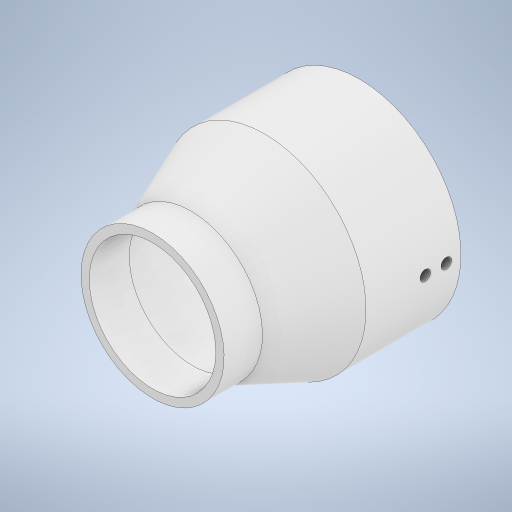
# Autodesk Inventor part: 2in to 4in Reducer
Saved by Autodesk Inventor 2023 (Build 270158030, 158C)
## iProperties
Created: 2022-10-01
Part Number: 2in to 4in Reducer
Material: PVC-Piping
Document SubType Name: Modeling
Designer: cjj5381
Density: 1.4 g/cm^3
Appearance: Smooth - White
Author: cjj5381
Autodesk Inventor part; units mm, degrees
ref_plane "YZ Plane" through (0, 0, 0) normal (1, 0, 0) x (0, 1, 0)
ref_plane "XZ Plane" through (0, 0, 0) normal (0, 1, 0) x (-1, 0, 0)
ref_plane "XY Plane" through (0, 0, 0) normal (0, 0, 1) x (1, 0, 0)
sketch "Sketch1" plane through (0, 0, 0) normal (1, 0, 0) x (0, 1, 0)
  line L0 (30.1625, 50.8) -> (30.1625, 31.75)
  line L1 (30.1625, 31.75) -> (44.45, -3.302)
  line L2 (44.45, -3.302) -> (44.45, -47.752)
  line L3 (0, 0) -> (0, 58.5884)
  line L4 (34.0741, 50.8) -> (34.0741, 32.5166)
  line L5 (34.0741, 32.5166) -> (48.3616, -2.5354)
  line L6 (48.3616, -2.5354) -> (48.3616, -47.752)
  line L7 (34.0741, 50.8) -> (30.1625, 50.8)
  line L8 (48.3616, -47.752) -> (44.45, -47.752)
  line L9 (0, 0) -> (18.7543, 0) construction
  dimension "d0" = 60.325
  dimension "d1" = 88.9
  dimension "d2" = 19.05
  dimension "d3" = 44.45
  dimension "d4" = 3.9116
  dimension "d5" = 98.552
  dimension "d6" = 50.8
  constraints: 20 end point, 3 parallel, 2 horizontal, 2 vertical, 2 other
  measures "d0" diameter of L0 L3
  measures "d1" diameter of L2 L3
  measures "d2" distance of L0.start L0.end
  measures "d3" distance of L1.end L2.end
  measures "d4" distance between parallel lines of L0 L4
  measures "d5" vertical distance of L2.end L0.start
  measures "d6" distance from line of L0.start L9
revolve "Revolution1" add sketch "Sketch1" angle 360 about axis through (0, 0, 0) along (0, 0, 1)
sketch "Sketch3" plane through (0, 0, 0) normal (1, 0, 0) x (0, 1, 0)
  circle A0 centre (0, -40.752) radius 2.5
  circle A1 centre (0, -30.752) radius 2.5
  line L0 (44.45, -47.752) -> (-44.45, -47.752) projected
  point P0 (0, 0)
  dimension "d8" = 5
  dimension "d9" = 5
  dimension "d10" = 7
  dimension "d11" = 10
  constraints: 2 centre point
  measures "d8" diameter of A0
  measures "d9" diameter of A1
  measures "d10" distance from line of L0 A0.centre
  measures "d11" distance of A0.centre A1.centre
extrude "Extrusion1" cut sketch "Sketch3" along normal through all both and the other way through all
body "Solid1"
